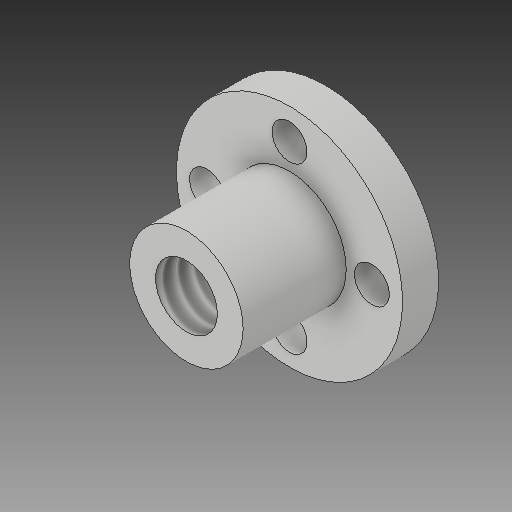
# Autodesk Inventor part: Brass-Nut
Saved by Autodesk Inventor 2018 (Build 220112000, 112)
## iProperties
Created: 2016-07-12
Part Number: Brass-Nut
Material: Generic
Document SubType Name: Modeling
Designer: joshmamo
Density: 1 g/cm^3
Appearance: Default
Author: joshmamo
Autodesk Inventor part; units mm, degrees
ref_plane "YZ Plane" through (0, 0, 0) normal (1, 0, 0) x (0, 1, 0)
ref_plane "XZ Plane" through (0, 0, 0) normal (0, 1, 0) x (-1, 0, 0)
ref_plane "XY Plane" through (0, 0, 0) normal (0, 0, 1) x (1, 0, 0)
sketch "Sketch1" plane through (0, 0, 0) normal (0, 0, 1) x (1, 0, 0)
  circle A0 centre (-24.8164, 12.4312) radius 5.5 projected
  circle A1 centre (-24.8164, 12.4312) radius 10.965
  circle A2 centre (-24.8164, 12.4312) radius 5.08
  point P0 (0, 0)
  dimension "d0" = 21.93
  dimension "d1" = 10.16
  constraints: 2 centre point, 2 coincident
  measures "d0" diameter of A1
  measures "d1" diameter of A2
extrude "Extrusion1" add sketch "Sketch1" along normal blind 3.5 contours A1
sketch "Sketch2" plane through (-24.8164, 12.4312, 3.5) normal (0, 0, 1) x (1, 0, 0)
  circle A0 centre (0, 0) radius 3
  circle A1 centre (0, 0) radius 5.5
  point P0 (24.8164, -12.4312)
  dimension "d4" = 6
  constraints: 2 centre point, 1 coincident
  measures "d4" diameter of A0
extrude "Extrusion2" add sketch "Sketch2" along normal blind 10
sketch "Sketch3" plane through (-24.8164, 12.4312, 3.5) normal (0, 0, 1) x (1, 0, 0)
  circle A0 centre (-8, -0.0188) radius 1.7 projected
  circle A1 centre (0, -8.0188) radius 1.7 projected
  circle A2 centre (8, -0.0188) radius 1.7 projected
  circle A3 centre (0, 7.9812) radius 1.7 projected
  point P0 (24.8164, -12.4312)
extrude "Extrusion3" cut sketch "Sketch3" against normal blind 10
thread "Thread1" size "M10x1.5" class "6H" standard "ANSI Metric M Profile" full length
body "Solid1"
